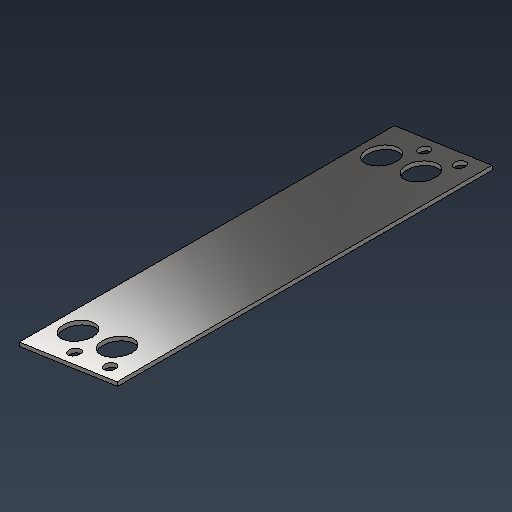
# Autodesk Inventor part: SteelFront
Saved by Autodesk Inventor 2026.2 (Build 302298010, 298A)
## iProperties
Created: 2026-04-07
Part Number: SteelFront
Material: Steel, Alloy
Document SubType Name: Modeling
Designer: szymo
Density: 7.73 g/cm^3
Appearance: Semi-Polished(2)
Mass: 18.6952 g
Surface Area: 52.2825 cm^2
Volume: 2.41853 cm^3
Author: szymo
Autodesk Inventor part; units mm, degrees
ref_plane "YZ Plane" through (0, 0, 0) normal (1, 0, 0) x (0, 1, 0)
ref_plane "XZ Plane" through (0, 0, 0) normal (0, 1, 0) x (-1, 0, 0)
ref_plane "XY Plane" through (0, 0, 0) normal (0, 0, 1) x (1, 0, 0)
sketch "Sketch1" plane through (0, 0, 0) normal (0, 0, 1) x (1, 0, 0)
  line L0 (0, -95.5) -> (0, -82.632) construction
  line L1 (3, -82.632) -> (3, -91) construction
  line L2 (3, -91) -> (4.5, -91) construction
  line L3 (4.5, -91) -> (0, -95.5) construction
  circle A0 centre (14.5, -55.2958) radius 14.5 construction
  line L4 (3.3461, -90.8) -> (29.4, -86.9522)
  line L5 (29.4, -86.9522) -> (29.2539, -85.963)
  line L6 (29.2539, -85.963) -> (3.2, -89.8107)
  line L7 (3.2, -89.8107) -> (3.3461, -90.8)
  line L8 (29.4, -86.9522) -> (29.4, -70.3377) construction
  line L9 (27, -86.2958) -> (6.5, -86.2958) projected
  line L10 (6.5, -86.2958) -> (6.5, -69.7958) projected
  line L11 (27, -69.7958) -> (6.5, -69.7958) projected
  line L12 (27, -86.2958) -> (27, -69.7958) projected
  line L13 (0, -82.632) -> (3, -82.632) projected
  point P0 (2.5, -82.632)
  dimension "d0" = 1
  dimension "d1" = 0.2
  dimension "d2" = 0.2
  dimension "d3" = 0.4
  dimension "d4" = 0
  constraints: 10 end point, 2 parallel, 1 perpendicular, 1 vertical
  measures "d0" distance between parallel lines of L6 L4
  measures "d1" distance from line of L1 L6.end
  measures "d2" distance from line of L2 L4.start
  measures "d3" distance edge to line of A0 L8
  measures "d4" distance from line of L6 L9.start
extrude "Extrusion1" add sketch "Sketch1" along normal mid plane 100 contours L7 L6 L5 L4
sketch "Sketch2" plane through (29.4, -86.9522, -50) normal (0.1460998, -0.9892699, 0) x (0.9892699, 0.1460998, 0)
  line L0 (-23.5061, 15.5) -> (-23.5061, 84.5) projected
  line L1 (-26.5387, 0) -> (-26.5387, 100) projected
  circle A0 centre (-5.2783, 96.6469) radius 1.5
  circle A1 centre (-14.8697, 96.6469) radius 1.5
  circle A2 centre (-14.8697, 3.3531) radius 1.5
  circle A3 centre (-5.2783, 3.3531) radius 1.5
  circle A4 centre (-9.5918, 90.5) radius 4
  circle A5 centre (-20.1476, 90.5) radius 4
  circle A6 centre (-9.5918, 9.5) radius 4
  circle A7 centre (-20.1476, 9.5) radius 4
  circle A8 centre (-14.8697, 96.6469) radius 2.25 projected
  circle A9 centre (-5.2783, 96.6469) radius 2.25 projected
  ellipse E0 centre (-20.1476, 90.5) end of major axis (-15.6193, 90.5) minor radius 4.5 (-16.2241, 92.7467) -> (-16.2241, 88.2533) ccw projected
  line L2 (-16.2241, 92.7467) -> (-13.5153, 92.7467) projected
  ellipse E1 centre (-9.5918, 90.5) end of major axis (-5.0635, 90.5) minor radius 4.5 (-13.5153, 88.2533) -> (-13.5153, 92.7467) ccw projected
  line L3 (-13.5153, 88.2533) -> (-16.2241, 88.2533) projected
  circle A10 centre (-14.8697, 3.3531) radius 2.25 projected
  circle A11 centre (-5.2783, 3.3531) radius 2.25 projected
  ellipse E2 centre (-20.1476, 9.5) end of major axis (-15.6193, 9.5) minor radius 4.5 (-16.2241, 11.7467) -> (-16.2241, 7.2533) ccw projected
  line L4 (-16.2241, 11.7467) -> (-13.5153, 11.7467) projected
  ellipse E3 centre (-9.5918, 9.5) end of major axis (-5.0635, 9.5) minor radius 4.5 (-13.5153, 7.2533) -> (-13.5153, 11.7467) ccw projected
  line L5 (-13.5153, 7.2533) -> (-16.2241, 7.2533) projected
  line L6 (-2.2783, 84.5) -> (-23.5061, 84.5) projected
  line L7 (-2.2783, 84.5) -> (-2.2783, 100) projected
  line L8 (-2.2783, 100) -> (-26.5387, 100) projected
  line L9 (-2.2783, 0) -> (-26.5387, 0) projected
  line L10 (-2.2783, 15.5) -> (-2.2783, 0) projected
  line L11 (-2.2783, 15.5) -> (-23.5061, 15.5) projected
  point P0 (-16.3808, 50)
  point P1 (-13.5515, 92.7467)
  point P2 (-13.5515, 88.2533)
  point P3 (-13.5515, 11.7467)
  point P4 (-13.5515, 7.2533)
  point P5 (-23.4601, 15.5)
  point P6 (-23.4601, 84.5)
  point P7 (-26.484, 0)
  point P8 (-26.484, 100)
  point P9 (-16.2089, 88.2533)
  point P10 (-16.2089, 92.7467)
  point P11 (-16.2089, 7.2533)
  point P12 (-16.2089, 11.7467)
  point P13 (-2.2926, 84.5)
  point P14 (-2.2926, 100)
  point P15 (-2.2926, 0)
  point P16 (-2.2926, 15.5)
  point P17 (-13.5305, 92.7467)
  point P18 (-13.5305, 88.2533)
  point P19 (-13.5305, 11.7467)
  point P20 (-13.5305, 7.2533)
  point P21 (-23.4988, 15.5)
  point P22 (-23.4988, 84.5)
  point P23 (-16.2214, 88.2533)
  point P24 (-16.2214, 92.7467)
  point P25 (-16.2214, 7.2533)
  point P26 (-16.2214, 11.7467)
  point P27 (-2.2803, 84.5)
  point P28 (-2.2803, 100)
  point P29 (-2.2803, 0)
  point P30 (-2.2803, 15.5)
  dimension "d7" = 3
  dimension "d8" = 3
  dimension "d9" = 3
  dimension "d10" = 3
  dimension "d13" = 8
  dimension "d14" = 8
  dimension "d15" = 8
  dimension "d16" = 8
  constraints: 8 centre point, 4 other
  measures "d7" diameter of A0
  measures "d8" diameter of A1
  measures "d9" diameter of A2
  measures "d10" diameter of A3
  measures "d13" diameter of A4
  measures "d14" diameter of A5
  measures "d15" diameter of A7
  measures "d16" diameter of A6
extrude "Extrusion2" cut sketch "Sketch2" against normal through all contours A0 | A1 | A2 | A3 | A4 | A5 | A6 | A7
equation "\"d14\" = d13"
equation "\"d15\" = d13"
equation "\"d16\" = d13"
body "Solid1"
